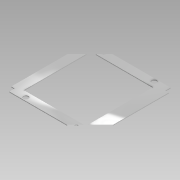
# Autodesk Inventor part: Carriage Sheet
Saved by Autodesk Inventor 2016 (Build 200138000, 138)
## iProperties
Created: 2017-05-17
Part Number: Carriage Sheet
Material: Generic
Document SubType Name: Modeling
Designer: 31745
Density: 1 g/cm^3
Appearance: Aluminum - Dark
Author: 31745
Autodesk Inventor part; units mm, degrees
ref_plane "YZ Plane" through (0, 0, 0) normal (1, 0, 0) x (0, 1, 0)
ref_plane "XZ Plane" through (0, 0, 0) normal (0, 1, 0) x (-1, 0, 0)
ref_plane "XY Plane" through (0, 0, 0) normal (0, 0, 1) x (1, 0, 0)
sketch "Sketch1" plane through (0, 0, 0) normal (0, 1, 0) x (-1, 0, 0)
  line L0 (0, 0) -> (-254, 0)
  line L1 (-254, 0) -> (-254, -254)
  line L2 (-254, -254) -> (0, -254)
  line L3 (0, -254) -> (0, 0)
  line L4 (0, -15.875) -> (-10.287, -15.875)
  line L5 (-10.287, -15.875) -> (-10.287, 0)
  line L6 (-243.713, 0) -> (-243.713, -15.875)
  line L7 (-243.713, -15.875) -> (-254, -15.875)
  line L8 (-243.713, -254) -> (-243.713, -238.125)
  line L9 (-243.713, -238.125) -> (-254, -238.125)
  line L10 (-10.287, -254) -> (-10.287, -238.125)
  line L11 (-10.287, -238.125) -> (0, -238.125)
  dimension "d0" = 254
  dimension "d1" = 254
  dimension "d14" = 10.287
  dimension "d15" = 10.287
  dimension "d16" = 15.875
  dimension "d17" = 15.875
  constraints: 24 end point, 12 point on line, 5 perpendicular, 2 horizontal, 2 horizontal alignment, 2 parallel, 1 vertical, 1 vertical alignment
  measures "d0" distance of L2.end L1.end
  measures "d1" distance of L1.end L0.end
  measures "d14" distance of L4.start L4.end
  measures "d15" distance of L6.end L7.end
  measures "d16" distance of L10.start L10.end
  measures "d17" distance of L4.end L5.end
extrude "Extrusion1" add sketch "Sketch1" along normal blind 2.286 contours L5 L4 L3 L11 L10 L2 L8 L9 L1 L7 L6 L0
sketch "Sketch2" plane through (0, 2.286, 0) normal (0, 1, 0) x (1, 0, 0)
  line L0 (28.575, 25.4) -> (211.9884, 25.4)
  line L1 (211.9884, 25.4) -> (211.9884, 228.6)
  line L2 (211.9884, 228.6) -> (28.575, 228.6)
  line L3 (28.575, 228.6) -> (28.575, 25.4)
  line L4 (0, 15.875) -> (10.287, 15.875) projected
  line L5 (10.287, 15.875) -> (10.287, 0) projected
  line L6 (10.287, 0) -> (243.713, 0) projected
  line L7 (243.713, 0) -> (243.713, 15.875) projected
  line L8 (243.713, 15.875) -> (254, 15.875) projected
  line L9 (254, 15.875) -> (254, 238.125) projected
  line L10 (254, 238.125) -> (243.713, 238.125) projected
  line L11 (243.713, 238.125) -> (243.713, 254) projected
  line L12 (243.713, 254) -> (10.287, 254) projected
  line L13 (10.287, 254) -> (10.287, 238.125) projected
  line L14 (10.287, 238.125) -> (0, 238.125) projected
  line L15 (0, 238.125) -> (0, 15.875) projected
  point P0 (0, 0)
  point P1 (127, 0)
  point P2 (0, 127)
  dimension "d9" = 203.2
  dimension "d28" = 42.0116
  dimension "d29" = 28.575
  constraints: 8 end point, 2 midpoint
  measures "d9" distance of L2.end L0.start
  measures "d28" distance between parallel lines of L9 L1
  measures "d29" distance between parallel lines of L15 L3
extrude "Extrusion2" cut sketch "Sketch2" against normal through all contours L3 L2 L1 L0
sketch "Sketch3" plane through (0, 2.286, 0) normal (0, 1, 0) x (1, 0, 0)
  circle A0 centre (50.8, 9.525) radius 4 projected
  circle A1 centre (203.2, 9.525) radius 4 projected
  circle A2 centre (203.2, 244.475) radius 4.2037 projected
  circle A3 centre (50.8, 244.475) radius 4.2037 projected
  point P0 (0, 0)
hole "Hole1" at (50.8, 2.286, -9.525) at (50.8, 2.286, -244.475) at (203.2, 2.286, -244.475) at (203.2, 2.286, -9.525) direction (0, -1, 0) diameter 15 end through all
chamfer "Chamfer1" distance 3.175 angle 45 1 edges at (0, 1.143, -238.125)
equation "\"d15\" = d14"
equation "\"d17\" = d16"
body "Solid1"
